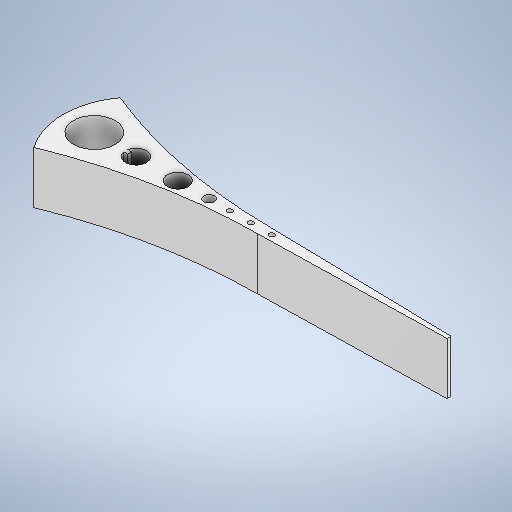
# Autodesk Inventor part: mover
Saved by Autodesk Inventor 2025.3 (Build 293356000, 356)
## iProperties
Created: 2026-03-18
Part Number: mover
Material: PC/ABS Plastic
Document SubType Name: Modeling
Designer: abdul
Density: 1.1 g/cm^3
Appearance: Smooth - White
Mass: 43.7804 g
Surface Area: 175.818 cm^2
Volume: 39.8004 cm^3
Author: abdul
## iProperties of the stored document mover_3DPrint.ipt
Created: 2026-04-12
Part Number: mover_3DPrint
Material: Generic
Document SubType Name: Modeling
Designer: kamal
Density: 1 g/cm^3
Appearance: Default
Author: kamal
Autodesk Inventor part; units mm, degrees
ref_plane "YZ Plane" through (0, 0, 0) normal (1, 0, 0) x (0, 1, 0)
ref_plane "XZ Plane" through (0, 0, 0) normal (0, 1, 0) x (-1, 0, 0)
ref_plane "XY Plane" through (0, 0, 0) normal (0, 0, 1) x (1, 0, 0)
sketch "Sketch3" plane through (0, 0, 0) normal (0, 1, 0) x (-1, 0, 0)
  circle A0 centre (0, 0) radius 39.5
  line L0 (0, 0) -> (-150, 0)
  line L1 (-150, 0) -> (-150, 25)
  line L2 (-150, 0) -> (-150, -25)
  line L3 (-150, 0) -> (-150, 1.869)
  line L4 (-150, 0) -> (32.5266, 22.4114) construction
  line L5 (-150, 0) -> (33.8973, 0) construction
  arc A1 (-61.0323, 2.8576) -> (32.5266, 22.4114) centre (-62.3689, 242.8539) ccw
  arc A2 (32.5266, -22.4114) -> (-61.0323, -2.8576) centre (-62.3689, -242.8539) ccw
  circle A3 centre (0, 0) radius 5
  line L6 (-150, 0.9345) -> (-100.7064, 2)
  line L7 (-150, -0.9345) -> (-61.0323, -2.8576)
  line L8 (-150, 0.9345) -> (-61.0323, 2.8576)
  point P0 (-150, -1.869)
  point P1 (-150, -6)
  point P2 (32.5266, -22.4114)
  point P3 (-100.7064, -2)
  point P4 (-39.3005, 3.9651)
  point P5 (-39.3005, -3.9651)
  point P6 (-150, 0.9345)
  dimension "d17" = 79
  dimension "d18" = 150
  dimension "d19" = 25
  dimension "d20" = 25
  dimension "d22" = 7
  dimension "d23" = 10
  dimension "d26" = 240
  dimension "d27" = 1.238
  dimension "d28" = 25.6262
  dimension "d29" = 50.7411
  dimension "d30" = 2
  dimension "d33" = 1.238
  constraints: 18 end point, 6 symmetric about line, 4 point on circle, 3 centre point, 2 coincident, 2 horizontal, 2 point on line, 2 vertical, 1 equal length, 1 midpoint, 4 other
  measures "d18" distance of L0.start L0.end
  measures "d19" distance of L0.end L1.end
  measures "d20" distance of L0.end L2.end
  measures "d22" angle of L5 L4
  measures "d23" diameter of A3
  measures "d26" radius of A1
  measures "d27" angle of L5 L6
  measures "d30" distance from line of L6.end L5
  measures "d33" angle of L0 L7
extrude "Extrusion2" add sketch "Sketch3" along normal blind 25 contours A0 A2 A1 | A0 L0 L1 L6 L8 A1 | A2 L7 L2 L0 A0
sketch "Sketch4" plane through (0, 25, 0) normal (0, 1, 0) x (1, 0, 0)
  arc A0 (-28.2743, -20.6292) -> (-28.2743, 20.6292) centre (0, 0) ccw construction
  arc A1 (61.0323, -2.8576) -> (-32.5266, -22.4114) centre (62.3689, -242.8539) ccw projected
  arc A2 (-32.5266, 22.4114) -> (61.0323, 2.8576) centre (62.3689, 242.8539) ccw projected
  arc A3 (-28.2743, 20.6292) -> (-28.2743, -20.6292) centre (0, 0) ccw
  arc A4 (-32.5266, 22.4114) -> (-32.5266, -22.4114) centre (0, 0) ccw projected
  dimension "d35" = 70
  constraints: 6 point on circle, 2 centre point, 1 coincident
  measures "d35" diameter of A0
extrude "Extrusion3" cut sketch "Sketch4" against normal through all
sketch "Sketch5" plane through (0, 25, 0) normal (0, 1, 0) x (1, 0, 0)
  circle A0 centre (0, 0) radius 5 projected
  line L0 (-3, 1) -> (-7, 1)
  line L1 (-7, 1) -> (-7, -1)
  line L2 (-7, -1) -> (-3, -1)
  line L3 (-3, -1) -> (-3, 1)
  line L4 (-3, 1) -> (-7, -1) construction
  line L5 (-7, 1) -> (-3, -1) construction
  point P0 (-5, 0)
  point P1 (-4.899, -1)
  point P2 (-4.899, 1)
  dimension "d42" = 5
  dimension "d43" = 2
  dimension "d44" = 4
  dimension "d45" = 3
  constraints: 12 end point, 2 midpoint, 2 parallel, 1 horizontal, 1 perpendicular
  measures "d42" distance of point (0, 0) point (-5, 0)
  measures "d43" distance of L0.end L1.end
  measures "d44" distance of L0.start L0.end
  measures "d45" distance from line of point (0, 0) L3
sketch "Sketch6" plane through (0, 25, 0) normal (0, 1, 0) x (1, 0, 0)
  arc A0 (-5, 0) -> (-5, 0) centre (0, 0) ccw projected
  line L0 (-7, 1) -> (-5, 1) projected
  line L1 (-5, -1) -> (-7, -1) projected
  line L2 (-7, -1) -> (-7, 1) projected
extrude "Extrusion5" add sketch "Sketch5" against normal blind 25 contours L0 L3 L2 A0 picked at (-3.6629, -0.1118)
sketch "Sketch8" plane through (0, 25, 0) normal (0, 1, 0) x (1, 0, 0)
  line L0 (0, 0) -> (5, 0) construction
  arc A0 (-4.899, -1) -> (-4.899, 1) centre (0, 0) ccw projected
  constraints: 2 end point, 1 horizontal, 1 point on circle
sketch "Sketch9" plane through (0, 25, 0) normal (0, 1, 0) x (1, 0, 0)
  arc A0 (-28.2743, 20.6292) -> (-28.2743, -20.6292) centre (0, 0) ccw projected
  arc A1 (-28.2743, 20.6292) -> (61.0323, 2.8576) centre (62.3689, 242.8539) ccw projected
  arc A2 (61.0323, -2.8576) -> (-28.2743, -20.6292) centre (62.3689, -242.8539) ccw projected
  line L0 (0, 0) -> (-20, 0) construction
  circle A3 centre (-20, 0) radius 10
  line L1 (0, 0) -> (20, 0) construction
  circle A4 centre (20, 0) radius 5
  line L2 (20, 0) -> (35, 0) construction
  circle A5 centre (35, 0) radius 2.5
  line L3 (35, 0) -> (45, 0) construction
  circle A6 centre (45, 0) radius 1.25
  line L4 (45, 0) -> (55, 0) construction
  circle A7 centre (55, 0) radius 1.25
  line L5 (55, 0) -> (65, 0) construction
  circle A8 centre (65, 0) radius 1.25
  dimension "d50" = 20
  dimension "d51" = 20
  dimension "d52" = 20
  dimension "d53" = 10
  dimension "d54" = 15
  dimension "d55" = 5
  dimension "d60" = 10
  dimension "d61" = 2.5
  dimension "d62" = 10
  dimension "d63" = 2.5
  dimension "d64" = 10
  dimension "d65" = 2.5
  constraints: 12 end point, 6 centre point, 6 coincident, 6 horizontal
  measures "d50" distance of L0.start L0.end
  measures "d51" diameter of A3
  measures "d52" distance of L0.start L1.end
  measures "d53" diameter of A4
  measures "d54" distance of L2.start L2.end
  measures "d55" diameter of A5
  measures "d60" distance of L3.start L3.end
  measures "d61" diameter of A6
  measures "d62" distance of L4.start L4.end
  measures "d63" diameter of A7
  measures "d64" distance of L5.start L5.end
  measures "d65" diameter of A8
extrude "Extrusion6" cut sketch "Sketch9" against normal through all
body "Solid2"
